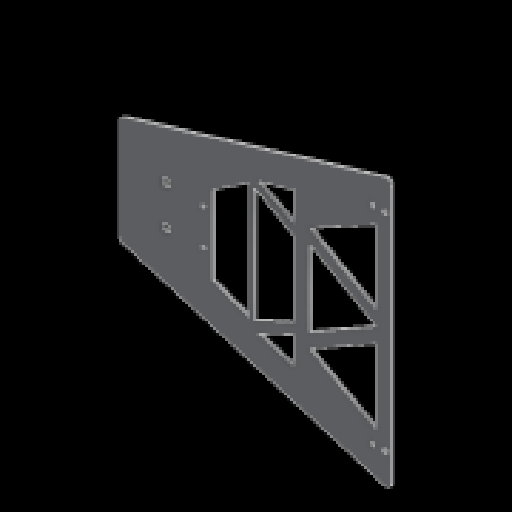
# Autodesk Inventor part: Part1
Saved by Autodesk Inventor 2025.2 (Build 292293000, 293)
## iProperties
Created: 2025-09-26
Part Number: Part1
Material: Generic
Document SubType Name: Sheet Metal
Designer: valer
Density: 1 g/cm^3
Sheet Metal Rule: Default
Appearance: Default
Author: valer
Autodesk Inventor part; units mm, degrees
ref_plane "YZ Plane" through (0, 0, 0) normal (1, 0, 0) x (0, 1, 0)
ref_plane "XZ Plane" through (0, 0, 0) normal (0, 1, 0) x (-1, 0, 0)
sketch "Base" plane through (0, 0, 0) normal (0, 0, 1) x (1, 0, 0)
  line L0 (-173.8499, -66.2658) -> (171.6188, -178.9186) construction
  line L1 (-9.525, -101.5493) -> (-9.525, 101.5493) construction
  line L2 (-9.525, 0) -> (-9.525, -119.85)
  line L3 (187.0398, -183.9472) -> (-9.525, -119.85)
  line L4 (187.0398, -183.9472) -> (187.0398, 0)
  line L5 (187.0398, 0) -> (-9.525, 0) construction
  line L6 (-9.525, 0) -> (-9.525, 119.85)
  line L7 (187.0398, 183.9472) -> (-9.525, 119.85)
  line L8 (187.0398, 183.9472) -> (187.0398, 0)
  point P0 (0, 0)
  point P1 (187.0398, -182.4643)
extrude "Plate1" add sketch "Base" along normal blind 3
sketch "MountHoles" plane through (0, 0, 0) normal (0, 0, -1) x (-1, 0, 0)
  line L0 (-179.0398, 172.9239) -> (1.525, 114.0441) construction
  circle A0 centre (-179.0398, 172.9239) radius 3
  circle A1 centre (1.525, 114.0441) radius 3
  line L1 (-226.3528, 0) -> (48.838, 0) construction
  circle A2 centre (-179.0398, -172.9239) radius 3
  circle A3 centre (1.525, -114.0441) radius 3
  line L2 (-187.0398, 183.9472) -> (9.525, 119.85) projected
  point P0 (0, 0)
  dimension "d2" = 6
  dimension "d3" = 6
  dimension "d45" = 8
  constraints: 4 centre point, 2 coincident, 2 end point, 2 symmetric about line, 2 other
  measures "d2" diameter of A0
  measures "d3" diameter of A1
  measures "d45" distance between parallel lines of L2 L0
extrude "MountHolesFeature" cut sketch "MountHoles" against normal blind 3
sketch "TorsoLiftMountHoles" plane through (0, 0, 3) normal (0, 0, 1) x (1, 0, 0)
  circle A0 centre (180.0398, -133.6037) radius 3 projected
  circle A1 centre (164.0398, -133.6037) radius 3 projected
  circle A2 centre (180.0398, 133.6037) radius 3 projected
  circle A3 centre (164.0398, 133.6037) radius 3 projected
  point P0 (0, 0)
extrude "TorsoLiftMountHolesFeature" cut sketch "TorsoLiftMountHoles" against normal blind 3
sketch "Continuation" plane through (0, 0, 0) normal (0, 0, -1) x (-1, 0, 0)
  line L0 (9.525, 119.85) -> (164.525, 69.3065)
  line L1 (-257.3528, 0) -> (234.838, 0) construction
  line L2 (9.525, -119.85) -> (164.525, -69.3065)
  line L3 (164.525, 69.3065) -> (164.525, -69.3065)
  line L4 (-187.0398, 183.9472) -> (9.525, 119.85)
  line L5 (9.525, 119.85) -> (9.525, -119.85)
  circle A0 centre (1.525, 114.0441) radius 3
  line L6 (1.525, 114.0441) -> (164.525, 60.8919) construction
  circle A1 centre (139.525, 69.0441) radius 3
  circle A2 centre (139.525, -69.0441) radius 3
  point P0 (0, 0)
  dimension "d46" = 155
  dimension "d47" = 25
  measures "d46" distance between parallel lines of L5 L3
  measures "d47" distance from line of L3 A1.centre
sheet face with bend "ContinuationFeature" sketch "Continuation" thickness 3 toward (0, 0, 1) bend radius 3 contours L0 L3 L2 L5
bend "Bend2"
fillet "OutsideFilletsFeature" radius 8 4 edges at (187.0398, -183.9472, 1.5) (187.0398, 183.9472, 1.5) (-164.525, 69.3065, 1.5) (-164.525, -69.3065, 1.5)
ref_plane "MidPlane" through (0, -71.2585, 3.048) normal (1, 0, 0) x (0, 0, -1)
sketch "BottomMountHoles" plane through (0, 0, 0) normal (0, 0, -1) x (-1, 0, 0)
  circle A0 centre (18.4607, -50.75) radius 2.75 projected
  circle A1 centre (18.4607, -8.25) radius 2.75 projected
  circle A2 centre (18.4607, 8.25) radius 2.75 projected
  circle A3 centre (18.4607, 50.75) radius 2.75 projected
  ellipse E0 centre (103.3601, -25.3391) end of major axis (108.1225, -25.3596) minor radius 4.7625 projected
  ellipse E1 centre (103.5793, 25.4605) end of major axis (108.3417, 25.4399) minor radius 4.7625 projected
  spline S0 degree 3 poles (-22.2189, -83.25) (-22.5891, -83.25) (-22.9886, -83.178) (-23.6929, -82.9105) (-24.0824, -82.71) (-24.7238, -82.1045) (-24.9548, -81.7839) (-25.3958, -80.8943) (-25.4483, -80.428) (-25.4764, -79.9859) (-25.4838, -79.5156) (-25.1415, -78.5243) (-24.922, -78.15) (-24.3999, -77.5609) (-24.0923, -77.3244) (-23.5146, -77.014) (-23.2534, -76.9113) (-22.8383, -76.8067) (-22.5689, -76.75) (-22.2189, -76.75) knots 0 0 0 0 0.111053 0.111053 0.202489 0.202489 0.273701 0.273701 0.38581 0.38581 0.497395 0.497395 0.578796 0.578796 0.654724 0.654724 0.709985 0.709985 0.740525 0.740525 0.740525 0.740525 construction
  arc A4 (-22.2189, 83.25) -> (-22.2189, 76.75) centre (-22.2189, 80) ccw construction
  arc A5 (-133.7189, -83.25) -> (-133.7189, -76.75) centre (-133.7189, -80) ccw construction
  spline S1 degree 3 poles (-133.7189, 83.25) (-133.3487, 83.25) (-132.9492, 83.178) (-132.2449, 82.9105) (-131.8554, 82.71) (-131.2141, 82.1045) (-130.983, 81.7839) (-130.542, 80.8943) (-130.4896, 80.428) (-130.4615, 79.9859) (-130.4541, 79.5156) (-130.7963, 78.5243) (-131.0158, 78.15) (-131.538, 77.5609) (-131.8456, 77.3244) (-132.4232, 77.014) (-132.6845, 76.9113) (-133.0996, 76.8067) (-133.3689, 76.75) (-133.7189, 76.75) knots 0 0 0 0 0.111053 0.111053 0.202489 0.202489 0.273701 0.273701 0.38581 0.38581 0.497395 0.497395 0.578796 0.578796 0.654725 0.654725 0.709986 0.709986 0.740527 0.740527 0.740527 0.740527 construction
  line L0 (167.4427, 0) -> (-246.1203, 0) construction
  point P0 (0, 0)
extrude "Cut8" cut sketch "BottomMountHoles" against normal blind 3 contours E0 | E1
delete faces "Delete1" heal yes whole lump no faces at (-139.4042, 72.0417, 2) (-4.5153, 113.8027, 2) (179.1606, 175.9215, 2) (179.1606, -169.9264, 2) (-4.5153, -114.2855, 2) (-139.4042, -66.0465, 2)
sketch "Sketch15" plane through (187.0398, -172.9239, 3) normal (0, 0, 1) x (1, 0, 0)
  line L0 (-346.045, 244.0304) -> (-10.4802, 353.4537) projected
  line L1 (-346.045, 244.0304) -> (-0.3836, 348.2954)
  line L2 (-423.7471, 172.9239) -> (72.8866, 172.9239) construction
  line L3 (0, 345.8479) -> (0, 0) projected
  arc A0 (0, 345.8479) -> (-10.4802, 353.4537) centre (-8, 345.8479) ccw projected
  arc A1 (-346.045, 244.0304) -> (-351.5648, 236.4246) centre (-343.5648, 236.4246) ccw projected
  line L4 (-351.5648, 109.4233) -> (-351.5648, 236.4246) projected
  line L5 (-346.045, 101.8175) -> (-0.3836, -2.4475)
  arc A2 (-10.4802, -7.6058) -> (0, 0) centre (-8, 0) ccw projected
  line L6 (-10.4802, -7.6058) -> (-346.045, 101.8175) projected
  arc A3 (-351.5648, 109.4233) -> (-346.045, 101.8175) centre (-343.5648, 109.4233) ccw projected
  point P0 (-187.0398, 172.9239)
  dimension "d84" = 178.725
  constraints: 4 end point, 2 symmetric about line, 1 point on circle
  measures "d84" angle of L0 L1
extrude "AdjustToProductionFeature" cut sketch "Sketch15" against normal blind 3 contours L0 A0 L1 | L5 A2 L6
delete faces "Delete2" heal yes whole lump no faces at (187.0208, 173.4763, 1) (187.0208, -173.4763, 2)
fillet "Fillet5" radius 6 2 edges at (187.0398, 175.4872, 1.5) (187.0398, -175.4872, 1.5)
sketch "ContactorMount" plane through (-164.525, -63.5006, 0) normal (0, 0, -1) x (-1, 0, 0)
  circle A0 centre (-109.3281, 40.5006) radius 2.25 projected
  circle A1 centre (-109.3281, 86.5006) radius 2.25 projected
  point P0 (-164.525, 63.5006)
extrude "Cut12" cut sketch "ContactorMount" against normal blind 3
sketch "Sketch19" plane through (-164.525, -63.5006, 0) normal (0, 0, -1) x (-1, 0, 0)
  line L0 (-332.5315, 63.5006) -> (-247.3998, 15.1574)
  line L1 (-247.3998, 15.1574) -> (-247.3998, 111.8439)
  line L2 (-247.3998, 111.8439) -> (-332.5315, 63.5006)
  line L3 (-332.5315, 82.9372) -> (-247.3998, 131.2805)
  line L4 (-247.3998, 131.2805) -> (-332.5315, 177.8709)
  line L5 (-332.5315, 177.8709) -> (-332.5315, 82.9372)
  line L6 (-351.5648, -103.9097) -> (-351.5648, 230.9109) projected
  line L7 (-351.5648, 63.5006) -> (0, 63.5006) construction
  line L8 (0, 0) -> (0, 127.0012) projected
  line L9 (-332.5315, 63.5006) -> (-332.5315, 82.9372) construction
  line L10 (-247.3998, 111.8439) -> (-247.3998, 131.2805) construction
  line L11 (-332.5315, 44.064) -> (-247.3998, -4.2792)
  line L12 (-247.3998, -4.2792) -> (-332.5315, -50.8696)
  line L13 (-332.5315, -50.8696) -> (-332.5315, 44.064)
  point P0 (-164.525, 63.5006)
  point P1 (-247.3998, 63.5006)
  constraints: 24 end point, 3 midpoint, 3 symmetric about line, 3 vertical, 2 parallel, 2 point on line
extrude "Cut13" cut sketch "Sketch19" against normal blind 3
fillet "Fillet8" radius 6 9 edges at (168.0065, -19.4366, 1.5) (168.0065, -114.3703, 1.5) (82.8748, -67.7798, 1.5) (82.8748, -48.3432, 1.5) (168.0065, 0, 1.5) (82.8748, 48.3432, 1.5) (168.0065, 19.4366, 1.5) (82.8748, 67.7798, 1.5) (168.0065, 114.3703, 1.5)
equation "\"d7\" = Thickness"
equation "\"d43\" = Thickness"
equation "\"d82\" = Thickness"
equation "\"d85\" = Thickness"
equation "\"d0\" = Thickness"
equation "\"d48\" = BendRadius"
equation "\"d49\" = BendReliefWidth"
equation "\"d51\" = MinimumRemnant"
equation "\"d50\" = BendReliefDepth"
equation "\"d52\" = TransitionRadius"
equation "\"BendRadius\" = Thickness"
equation "\"BendReliefWidth\" = Thickness"
equation "\"BendReliefDepth\" = 0.5 * Thickness"
equation "\"CornerReliefSize\" = 4 * Thickness"
equation "\"MinimumRemnant\" = 2 * Thickness"
equation "\"TransitionRadius\" = BendRadius"
equation "\"JacobiRadiusSize\" = BendRadius"
equation "\"GapSize\" = Thickness"
equation "\"Thickness\" = 3"
body "Solid1"
